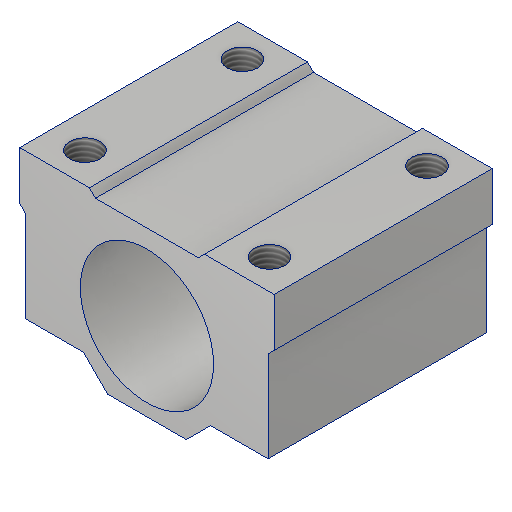
# Autodesk Inventor part: SC12UU
Saved by Autodesk Inventor 2022 (Build 260153000, 153)
## iProperties
Created: 2019-12-13
Part Number: SC12UU
Material: Generic
Document SubType Name: Modeling
Designer: nnico
Density: 1 g/cm^3
Appearance: Aluminum - Flat
Author: nnico
Autodesk Inventor part; units mm, degrees
ref_plane "YZ Plane" through (0, 0, 0) normal (1, 0, 0) x (0, 1, 0)
ref_plane "XZ Plane" through (0, 0, 0) normal (0, 1, 0) x (-1, 0, 0)
ref_plane "XY Plane" through (0, 0, 0) normal (0, 0, 1) x (1, 0, 0)
sketch "Sketch1" plane through (0, 0, 0) normal (0, 1, 0) x (-1, 0, 0)
  line L0 (21, -18) -> (-21, -18)
  line L1 (-21, -18) -> (-21, 18)
  line L2 (-21, 18) -> (21, 18)
  line L3 (21, 18) -> (21, -18)
  line L4 (0, -18) -> (0, 18) construction
  line L5 (21, 0) -> (-21, 0) construction
  point P0 (0, 0)
  point P1 (0, 0)
  dimension "d0" = 42
  dimension "d1" = 36
  constraints: 12 end point, 5 midpoint, 2 parallel, 1 coincident, 1 horizontal, 1 perpendicular
  measures "d0" distance of L0.start L0.end
  measures "d1" distance of L2.end L0.start
extrude "Extrusion1" add sketch "Sketch1" along normal blind 28
sketch "Sketch2" plane through (-21, 0, 18) normal (0, 0, 1) x (1, 0, 0)
  line L0 (42, 28) -> (0, 28) projected
  line L1 (21, 28) -> (21, 0) construction
  line L2 (0, 0) -> (0, 28) projected
  line L3 (0, 13) -> (42, 13) construction
  circle A0 centre (21, 13) radius 11
  dimension "d4" = 15
  dimension "d5" = 22
  constraints: 4 end point, 2 midpoint, 1 centre point, 1 horizontal, 1 point on line, 1 vertical
  measures "d4" distance of L0.start L3.end
  measures "d5" diameter of A0
extrude "Extrusion2" cut sketch "Sketch2" against normal up to next
sketch "Sketch3" plane through (0, 28, 0) normal (0, 1, 0) x (1, 0, 0)
  line L0 (-15.25, 13) -> (15.25, 13) construction
  line L1 (15.25, 13) -> (15.25, -13) construction
  line L2 (15.25, -13) -> (-15.25, -13) construction
  line L3 (-15.25, -13) -> (-15.25, 13) construction
  line L4 (0, 13) -> (0, -13) construction
  line L5 (-15.25, 0) -> (15.25, 0) construction
  circle A0 centre (-15.25, 13) radius 2.15
  circle A1 centre (-15.25, -13) radius 2.15
  circle A2 centre (15.25, 13) radius 2.15
  circle A3 centre (15.25, -13) radius 2.15
  point P0 (0, 0)
  point P1 (0, 0)
  dimension "d8" = 26
  dimension "d9" = 30.5
  dimension "d10" = 4.3
  dimension "d11" = 4.3
  dimension "d12" = 4.3
  dimension "d13" = 4.3
  constraints: 12 end point, 5 coincident, 5 midpoint, 4 centre point, 2 parallel, 1 horizontal, 1 perpendicular
  measures "d8" distance of L0.end L1.end
  measures "d9" distance of L0.start L0.end
  measures "d10" diameter of A0
  measures "d11" diameter of A1
  measures "d12" diameter of A2
  measures "d13" diameter of A3
extrude "Extrusion3" cut sketch "Sketch3" against normal up to next
sketch "Sketch4" plane through (0, 28, 0) normal (0, 1, 0) x (1, 0, 0)
  circle A0 centre (15.25, -13) radius 2.15 projected
  circle A1 centre (15.25, -13) radius 2.5
  circle A2 centre (-15.25, -13) radius 2.15 projected
  circle A3 centre (-15.25, -13) radius 2.5
  circle A4 centre (15.25, 13) radius 2.15 projected
  circle A5 centre (15.25, 13) radius 2.5
  circle A6 centre (-15.25, 13) radius 2.15 projected
  circle A7 centre (-15.25, 13) radius 2.5
  point P0 (0, 0)
  dimension "d16" = 5
  dimension "d17" = 5
  dimension "d18" = 5
  dimension "d19" = 5
  constraints: 4 centre point, 4 coincident
  measures "d16" diameter of A1
  measures "d17" diameter of A3
  measures "d18" diameter of A5
  measures "d19" diameter of A7
extrude "Extrusion5" cut sketch "Sketch4" against normal blind 12 contours A1 | A3 | A4 | A5 | A7
sketch "Sketch5" plane through (-21, 0, 18) normal (0, 0, 1) x (1, 0, 0)
  line L0 (0, 28) -> (42, 28) construction
  line L1 (21, 28) -> (21, 0) construction
  line L2 (42, 0) -> (0, 0) construction
  line L3 (0, 28) -> (0, 20)
  line L4 (0, 0) -> (0, 28) projected
  line L5 (21, 0) -> (14.5, 0)
  line L6 (10.5, 4) -> (14.5, 0)
  line L7 (0, 20) -> (1, 19)
  line L8 (1, 19) -> (1, 4)
  line L9 (1, 4) -> (10.5, 4)
  line L10 (0, 20) -> (0, 0)
  line L11 (14.5, 0) -> (0, 0)
  line L12 (0, 0) -> (42, 0) construction
  line L13 (42, 0) -> (42, 28)
  line L14 (31.5, 4) -> (27.5, 0)
  line L15 (42, 20) -> (41, 19)
  line L16 (41, 19) -> (41, 4)
  line L17 (41, 4) -> (31.5, 4)
  line L18 (27.5, 0) -> (42, 0)
  dimension "d27" = 8
  dimension "d28" = 9
  dimension "d29" = 135
  dimension "d35" = 9.5
  dimension "d43" = 135
  dimension "d44" = 24
  constraints: 32 end point, 7 symmetric about line, 4 point on line, 3 perpendicular, 1 collinear, 1 horizontal, 1 midpoint
  measures "d27" distance of L0.start L3.end
  measures "d28" distance from line of L0 L7.end
  measures "d29" angle of L3 L7
  measures "d35" distance of L8.end L6.start
  measures "d43" angle of L9 L6
  measures "d44" distance from line of L0 L8.end
extrude "Extrusion7" cut sketch "Sketch5" against normal up to next
sketch "Sketch6" plane through (0, 28, 0) normal (0, 1, 0) x (1, 0, 0)
  line L0 (6.5, -18) -> (10.5, -18) projected
  circle A0 centre (15.25, -13) radius 2.5 construction
  line L1 (15.25, -13) -> (15.25, -18) construction
  line L2 (-21, -18) -> (21, -18) construction
  line L3 (21, 18) -> (-21, 18) projected
  line L4 (9.5, 18) -> (-9.5, 18)
  line L5 (-9.5, 18) -> (-9.5, -18)
  line L6 (-9.5, -18) -> (9.5, -18)
  line L7 (9.5, -18) -> (9.5, 18)
  line L8 (0, -18) -> (0, 18) construction
  line L9 (0, 18) -> (0, -18) construction
  point P0 (0, 0)
  dimension "d36" = 5.75
  constraints: 14 end point, 4 midpoint, 3 point on line, 2 parallel, 2 perpendicular, 1 collinear, 1 horizontal, 1 vertical
  measures "d36" distance of L6.end L1.end
extrude "Extrusion8" cut sketch "Sketch6" against normal blind 1
sketch "Sketch7" plane through (6.5, 0, -18) normal (0, 0, -1) x (-1, 0, 0)
  line L0 (16, 27) -> (-3, 27) projected
  line L1 (-3, 28) -> (-14.5, 28) projected
  line L2 (-3, 27) -> (-3, 28)
  line L3 (-3, 27) -> (-2, 27)
  line L4 (-2, 27) -> (-3, 28)
  line L5 (-3, 27) -> (-3, 28) construction
  line L6 (27.5, 28) -> (16, 28) construction
  line L7 (-3, 28) -> (16, 28) construction
  line L8 (6.5, 28) -> (6.5, 27) construction
  line L9 (-3, 27) -> (16, 27)
  line L10 (16, 27) -> (16, 28)
  line L11 (15, 27) -> (16, 28)
  line L12 (15, 27) -> (16, 27) construction
  point P0 (6.5, 0)
  dimension "d39" = 1
  constraints: 18 end point, 3 symmetric about line, 2 midpoint, 2 point on line, 1 collinear, 1 horizontal, 1 vertical
  measures "d39" distance of L0.end L3.end
extrude "Extrusion9" add sketch "Sketch7" against normal blind 36
thread "Thread1" size "M5x0.8" class "6H" standard "ANSI Metric M Profile" full length
thread "Thread2" size "M5x0.8" class "6H" standard "ANSI Metric M Profile" full length
thread "Thread3" size "M5x0.8" class "6H" standard "ANSI Metric M Profile" full length
thread "Thread4" size "M5x0.8" class "6H" standard "ANSI Metric M Profile" full length
body "Solid1"
